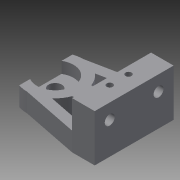
# Autodesk Inventor part: servo_clip_holder2
Saved by Autodesk Inventor 2015 (Build 190159000, 159)
## iProperties
Created: 2017-12-03
Part Number: servo_clip_holder2
Material: Generic
Document SubType Name: Modeling
Designer: Anshul
Density: 1 g/cm^3
Appearance: Default
Author: Anshul
Autodesk Inventor part; units mm, degrees
ref_plane "YZ Plane" through (0, 0, 0) normal (1, 0, 0) x (0, 1, 0)
ref_plane "XZ Plane" through (0, 0, 0) normal (0, 1, 0) x (-1, 0, 0)
ref_plane "XY Plane" through (0, 0, 0) normal (0, 0, 1) x (1, 0, 0)
sketch "Sketch1" plane through (0, 0, 0) normal (0, 1, 0) x (-1, 0, 0)
  line L0 (0, 0) -> (0, -42)
  line L1 (0, -42) -> (12, -42)
  line L2 (12, -42) -> (12, 0)
  line L3 (12, 0) -> (0, 0)
  line L4 (0, -21) -> (0, -26)
  line L5 (0, -21) -> (0, -16)
  line L6 (0, -16) -> (0, -19)
  line L7 (0, -16) -> (0, -13)
  line L8 (0, -26) -> (0, -23)
  line L9 (0, -26) -> (0, -29)
  line L10 (0, -29) -> (12, -29)
  line L11 (0, -13) -> (12, -13)
  line L12 (6.4, -16) -> (12, -16)
  line L13 (6.4, -26) -> (12, -26)
  line L14 (12, -16) -> (8, -16)
  circle A0 centre (8, -16) radius 1.6
  circle A1 centre (8, -26) radius 1.6
  line L15 (12, -26) -> (8, -26)
  dimension "d9" = 3.2
  dimension "d10" = 3.2
  dimension "d0" = 42
  dimension "d1" = 12
  dimension "d2" = 5
  dimension "d3" = 5
  dimension "d4" = 3
  dimension "d5" = 3
  dimension "d6" = 3
  dimension "d7" = 3
  dimension "d8" = 4
  constraints: 32 end point, 12 point on line, 6 perpendicular, 2 horizontal alignment, 1 coincident, 1 horizontal, 1 midpoint, 1 parallel, 1 vertical, 4 other
  measures "d0" distance of L0.start L0.end
  measures "d1" distance of L0.end L1.end
  measures "d2" distance of L4.start L4.end
  measures "d3" distance of L4.start L5.end
  measures "d4" distance of L5.end L6.end
  measures "d5" distance of L5.end L7.end
  measures "d6" distance of L4.end L8.end
  measures "d7" distance of L4.end L9.end
  measures "d8" distance of L12.end L14.end
extrude "Extrusion1" add sketch "Sketch1" along normal blind 15
sketch "Sketch2" plane through (0, 0, 0) normal (0, -1, 0) x (1, 0, 0)
  line L0 (-12, 0) -> (-12, -42)
  line L1 (-12, -42) -> (-12, 0) projected
  line L2 (-12, -21) -> (-42, -21)
  circle A0 centre (-42, -21) radius 3.5
  arc A1 (-47, -35.1421) -> (-47, -6.8579) centre (-42, -21) ccw
  line L3 (-42, -21) -> (-47, -21)
  line L4 (-47, -21) -> (-47, -35.1421)
  line L5 (-47, -21) -> (-47, -6.8579)
  line L6 (-42, -36) -> (-12, -42)
  line L7 (-42, -6) -> (-12, 0)
  line L8 (-12, -42) -> (0, -42)
  line L9 (0, -42) -> (0, 0)
  line L10 (0, 0) -> (0, -42) projected
  line L11 (0, 0) -> (-12, 0)
  circle A2 centre (-8, -16) radius 1.6 projected
  circle A3 centre (-8, -16) radius 1.6
  circle A4 centre (-8, -26) radius 1.6 projected
  circle A5 centre (-8, -26) radius 1.6
  line L12 (-12, -42) -> (-12, -36.5)
  line L13 (-12, 0) -> (-12, -5.5)
  line L14 (-17, -6.5) -> (-32.2985, -9.5597)
  line L15 (-32.2985, -32.4403) -> (-17, -35.5)
  circle A6 centre (-42, -21) radius 5
  line L16 (-12, -21) -> (-17, -21)
  line L17 (-17, -16) -> (-17, -6.5)
  line L18 (-17, -26) -> (-17, -35.5)
  line L19 (-42, -16) -> (-33.9223, -16)
  line L20 (-27.8579, -16) -> (-12, -16)
  line L21 (-42, -26) -> (-33.9223, -26)
  line L22 (-27.8579, -26) -> (-12, -26)
  arc A7 (-47, -29.3703) -> (-47, -12.6297) centre (-42, -21) ccw
  point P0 (-47, -12.9223)
  point P1 (-47, -29.0777)
  dimension "d13" = 30
  dimension "d14" = 7
  dimension "d16" = 30
  dimension "d17" = 5
  dimension "d30" = 5.5
  dimension "d31" = 5.5
  dimension "d32" = 10
  dimension "d33" = 5
  dimension "d36" = 19.5
  constraints: 42 end point, 13 point on line, 12 point on circle, 6 centre point, 5 coincident, 5 perpendicular, 4 parallel, 4 tangent, 3 horizontal, 2 collinear, 1 midpoint
  measures "d13" distance of L2.start L2.end
  measures "d14" diameter of A0
  measures "d16" diameter of A1
  measures "d17" distance of L3.start L3.end
  measures "d30" distance of L0.end L12.end
  measures "d31" distance of L0.start L13.end
  measures "d32" diameter of A6
  measures "d33" distance of L2.start L16.end
  measures "d36" diameter of A7
extrude "Extrusion2" add sketch "Sketch2" along normal blind 10 contours L11 L9 L8 L0 | L0 L20 L17 L14 A1 L7 | A1 L2 A7 L5 | L0 L2 A1 L20 | L14 L17 L20 A1 | L0 L22 A1 L2 | A7 L2 A6 L5 | L6 A1 L15 L18 L22 L0 | A1 L4 A7 L2 | A6 L2 A0 L3 | A6 L2 A7 L4 | L3 A0 L2 A6 | L18 L15 A1 L22
sketch "Sketch3" plane through (0, 15, 0) normal (1, 0, 0) x (0, 0, -1)
  line L0 (0, -15) -> (42, -15)
  line L1 (42, -15) -> (0, -15) projected
  line L2 (21, -15) -> (34, -15)
  line L3 (34, -15) -> (34, -8)
  line L4 (21, -15) -> (8, -15)
  line L5 (8, -15) -> (8, -8)
  circle A0 centre (8, -8) radius 2.65
  circle A1 centre (34, -8) radius 2.65
  dimension "d22" = 13
  dimension "d23" = 7
  dimension "d24" = 13
  dimension "d25" = 7
  dimension "d26" = 5.3
  dimension "d27" = 5.3
  constraints: 10 end point, 2 centre point, 2 coincident, 2 perpendicular, 2 point on line, 1 horizontal, 1 midpoint
  measures "d22" distance of L2.start L2.end
  measures "d23" distance of L2.end L3.end
  measures "d24" distance of L2.start L4.end
  measures "d25" distance of L4.end L5.end
  measures "d26" diameter of A0
  measures "d27" diameter of A1
extrude "Extrusion4" cut sketch "Sketch3" against normal blind 15
extrude "Extrusion5" cut sketch "Sketch2" along normal blind 15 contours L14 L17 L20 A1 | L18 L15 A1 L22
extrude "Extrusion6" cut sketch "Sketch2" along normal blind 6 contours A7 L2 A6 L5 | A6 L2 A0 L3 | A6 L2 A7 L4 | L3 A0 L2 A6
body "Solid1"
